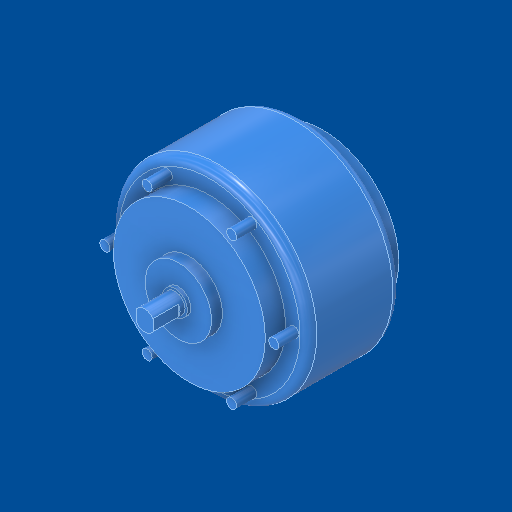
# Autodesk Inventor part: movero
Saved by Autodesk Inventor 2022.2 (Build 262287000, 287)
## iProperties
Created: 2017-11-21
Part Number: movero
Material: 一般
Document SubType Name: Modeling
Designer: gisen
Density: 2.885 g/cm^3
Appearance: シアン
Mass: 2200 g
Surface Area: 513.983 cm^2
Volume: 762.565 cm^3
Author: gisen
Autodesk Inventor part; units mm, degrees
ref_plane "YZ Plane" through (0, 0, 0) normal (1, 0, 0) x (0, 1, 0)
ref_plane "XZ Plane" through (0, 0, 0) normal (0, 1, 0) x (-1, 0, 0)
ref_plane "XY Plane" through (0, 0, 0) normal (0, 0, 1) x (1, 0, 0)
sketch "スケッチ1" plane through (0, 0, 0) normal (0, 0, 1) x (1, 0, 0)
  circle A0 centre (0, 0) radius 6
  dimension "d0" = 12
  constraints: 1 centre point, 1 coincident
  measures "d0" diameter of A0
extrude "押し出し1" add sketch "スケッチ1" along normal mid plane 132
sketch "スケッチ2" plane through (0, 0, 0) normal (0, 0, 1) x (1, 0, 0)
  circle A0 centre (0, 0) radius 6 construction
  circle A1 centre (0, 0) radius 7.4
  dimension "d3" = 14.8
  constraints: 1 centre point, 1 coincident
  measures "d3" diameter of A1
extrude "押し出し2" add sketch "スケッチ2" along normal mid plane 96
sketch "スケッチ3" plane through (0, 0, 0) normal (0, 0, 1) x (1, 0, 0)
  circle A0 centre (0, 0) radius 6 projected
  circle A1 centre (0, 0) radius 19.65
  dimension "d6" = 39.3
  constraints: 1 centre point, 1 coincident
  measures "d6" diameter of A1
extrude "押し出し3" add sketch "スケッチ3" along normal mid plane 92
sketch "スケッチ4" plane through (0, 0, 0) normal (0, 0, 1) x (1, 0, 0)
  circle A0 centre (0, 0) radius 45
  dimension "d9" = 90
  constraints: 1 centre point, 1 coincident
  measures "d9" diameter of A0
extrude "押し出し4" add sketch "スケッチ4" along normal mid plane 79
sketch "スケッチ5" plane through (0, 0, 0) normal (0, 0, 1) x (1, 0, 0)
  circle A0 centre (0, 0) radius 58.5
  dimension "d12" = 117
  constraints: 1 centre point, 1 coincident
  measures "d12" diameter of A0
extrude "押し出し5" add sketch "スケッチ5" along normal mid plane 55
fillet "フィレット1" radius 5 2 edges at (-58.5, 0, 27.5) (-58.5, 0, -27.5)
sketch "スケッチ6" plane through (0, 0, 39.5) normal (0, 0, 1) x (1, 0, 0)
  circle A0 centre (0, 0) radius 50 construction
  circle A1 centre (50, 0) radius 3
  circle A2 centre (25, 43.3013) radius 3
  circle A3 centre (-25, 43.3013) radius 3
  circle A4 centre (-50, 0) radius 3
  circle A5 centre (-25, -43.3013) radius 3
  circle A6 centre (25, -43.3013) radius 3
  dimension "d16" = 100
  dimension "d17" = 6
  dimension "d20" = 360
  constraints: 6 centre point, 1 coincident, 1 horizontal alignment, 15 other
  measures "d17" diameter of A1
extrude "押し出し6" add sketch "スケッチ6" against normal up to surface (12 mm away)
sketch "スケッチ7" plane through (0, 0, 66) normal (0, 0, 1) x (1, 0, 0)
  circle A0 centre (0, 0) radius 6 projected
  line L0 (-5, 3.3166) -> (-5, -3.3166)
  circle A1 centre (0, 0) radius 6 projected
  line L1 (5, 3.3166) -> (5, -3.3166)
  dimension "d24" = 5
  dimension "d25" = 5
  constraints: 4 end point, 3 point on circle, 1 parallel, 1 vertical, 2 other
  measures "d24" distance from line of point (0, 0) L0
  measures "d25" distance from line of L1 point (0, 0)
extrude "押し出し7" cut sketch "スケッチ7" against normal blind 15 contours A0 L1 | L0 A0
